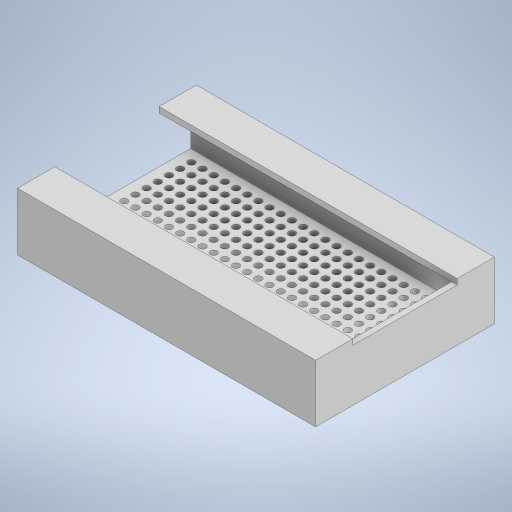
# Autodesk Inventor part: support batterie
Saved by Autodesk Inventor 2024 (Build 280153000, 153)
## iProperties
Created: 2024-02-10
Part Number: support batterie
Material: Generic
Document SubType Name: Modeling
Designer: Pooo
Density: 1 g/cm^3
Appearance: Default
Author: Pooo
Autodesk Inventor part; units mm, degrees
ref_plane "YZ Plane" through (0, 0, 0) normal (1, 0, 0) x (0, 1, 0)
ref_plane "XZ Plane" through (0, 0, 0) normal (0, 1, 0) x (-1, 0, 0)
ref_plane "XY Plane" through (0, 0, 0) normal (0, 0, 1) x (1, 0, 0)
sketch "Sketch1" plane through (0, 0, 0) normal (0, 1, 0) x (-1, 0, 0)
  point P0 (0, 0)
sketch "Sketch2" plane through (0, 0, 0) normal (0, 1, 0) x (-1, 0, 0)
  line L0 (43.1586, 43.7586) -> (-113.8414, 43.7586)
  line L1 (-113.8414, 43.7586) -> (-113.8414, -46.2414)
  line L2 (-113.8414, -46.2414) -> (43.1586, -46.2414)
  line L3 (43.1586, -46.2414) -> (43.1586, 43.7586)
  line L4 (43.1586, -46.2414) -> (-113.8414, -46.2414)
  line L5 (-113.8414, -46.2414) -> (-113.8414, -49.2414)
  line L6 (-113.8414, -49.2414) -> (43.1586, -49.2414)
  line L7 (43.1586, -49.2414) -> (43.1586, -46.2414)
  line L8 (43.1586, 43.7586) -> (-113.8414, 43.7586)
  line L9 (-113.8414, 43.7586) -> (-113.8414, 46.7586)
  line L10 (-113.8414, 46.7586) -> (43.1586, 46.7586)
  line L11 (43.1586, 46.7586) -> (43.1586, 43.7586)
  line L12 (-113.8414, 46.7586) -> (-116.8414, 46.7586)
  line L13 (-116.8414, 46.7586) -> (-116.8414, -49.2414)
  line L14 (-116.8414, -49.2414) -> (-113.8414, -49.2414)
  line L15 (-113.8414, -49.2414) -> (-113.8414, 46.7586)
  point P0 (0, 0)
  dimension "d0" = 90
  dimension "d1" = 157
  dimension "d2" = 3
  dimension "d3" = 3
  dimension "d4" = 3
  constraints: 32 end point, 8 parallel, 4 horizontal, 4 perpendicular
  measures "d0" distance of L2.end L0.start
  measures "d1" distance of L1.end L2.end
  measures "d2" distance of L4.end L5.end
  measures "d3" distance of L8.end L9.end
  measures "d4" distance of L14.end L13.end
extrude "Extrusion1" add sketch "Sketch2" along normal blind 3
sketch "Sketch3" plane through (0, 3, 0) normal (0, 1, 0) x (1, 0, 0)
  line L0 (-43.1586, -46.7586) -> (116.8414, -46.7586) projected
  line L1 (116.8414, -46.7586) -> (116.8414, 49.2414) projected
  line L2 (-43.1586, -46.7586) -> (116.8414, -46.7586)
  line L3 (116.8414, -46.7586) -> (116.8414, -43.7586)
  line L4 (116.8414, -43.7586) -> (-43.1586, -43.7586)
  line L5 (-43.1586, -43.7586) -> (-43.1586, -46.7586)
  line L6 (116.8414, 49.2414) -> (-43.1586, 49.2414) projected
  line L7 (-43.1586, 49.2414) -> (116.8414, 49.2414)
  line L8 (116.8414, 49.2414) -> (116.8414, 46.2414)
  line L9 (116.8414, 46.2414) -> (-43.1586, 46.2414)
  line L10 (-43.1586, 46.2414) -> (-43.1586, 49.2414)
  line L11 (116.8414, -43.7586) -> (113.8414, -43.7586)
  line L12 (113.8414, -43.7586) -> (113.8414, 46.2414)
  line L13 (113.8414, 46.2414) -> (116.8414, 46.2414)
  line L14 (116.8414, 46.2414) -> (116.8414, -43.7586)
  point P0 (0, 0)
  dimension "d7" = 3
  dimension "d8" = 3
  dimension "d9" = 3
  constraints: 24 end point, 6 parallel, 3 horizontal, 3 perpendicular, 3 point on line
  measures "d7" distance of L3.end L2.end
  measures "d8" distance of L7.end L8.end
  measures "d9" distance of L12.end L13.end
sketch "Sketch5" plane through (0, 3, 0) normal (0, 1, 0) x (1, 0, 0)
  circle A0 centre (-36.5125, -38.1) radius 1.85
  line L0 (-36.5125, -38.1) -> (-35.8777, -38.1)
  line L1 (-36.5125, -38.1) -> (-36.5125, -37.4601)
  circle A1 centre (-36.5125, -32.1) radius 1.85
  circle A2 centre (-36.5125, -26.1) radius 1.85
  circle A3 centre (-36.5125, -20.1) radius 1.85
  circle A4 centre (-36.5125, -14.1) radius 1.85
  circle A5 centre (-36.5125, -8.1) radius 1.85
  circle A6 centre (-36.5125, -2.1) radius 1.85
  circle A7 centre (-36.5125, 3.9) radius 1.85
  circle A8 centre (-36.5125, 9.9) radius 1.85
  circle A9 centre (-36.5125, 15.9) radius 1.85
  circle A10 centre (-36.5125, 21.9) radius 1.85
  circle A11 centre (-36.5125, 27.9) radius 1.85
  circle A12 centre (-36.5125, 33.9) radius 1.85
  circle A13 centre (-36.5125, 39.9) radius 1.85
  circle A14 centre (-30.5125, -38.1) radius 1.85
  circle A15 centre (-30.5125, -32.1) radius 1.85
  circle A16 centre (-30.5125, -26.1) radius 1.85
  circle A17 centre (-30.5125, -20.1) radius 1.85
  circle A18 centre (-30.5125, -14.1) radius 1.85
  circle A19 centre (-30.5125, -8.1) radius 1.85
  circle A20 centre (-30.5125, -2.1) radius 1.85
  circle A21 centre (-30.5125, 3.9) radius 1.85
  circle A22 centre (-30.5125, 9.9) radius 1.85
  circle A23 centre (-30.5125, 15.9) radius 1.85
  circle A24 centre (-30.5125, 21.9) radius 1.85
  circle A25 centre (-30.5125, 27.9) radius 1.85
  circle A26 centre (-30.5125, 33.9) radius 1.85
  circle A27 centre (-30.5125, 39.9) radius 1.85
  circle A28 centre (-24.5125, -38.1) radius 1.85
  circle A29 centre (-24.5125, -32.1) radius 1.85
  circle A30 centre (-24.5125, -26.1) radius 1.85
  circle A31 centre (-24.5125, -20.1) radius 1.85
  circle A32 centre (-24.5125, -14.1) radius 1.85
  circle A33 centre (-24.5125, -8.1) radius 1.85
  circle A34 centre (-24.5125, -2.1) radius 1.85
  circle A35 centre (-24.5125, 3.9) radius 1.85
  circle A36 centre (-24.5125, 9.9) radius 1.85
  circle A37 centre (-24.5125, 15.9) radius 1.85
  circle A38 centre (-24.5125, 21.9) radius 1.85
  circle A39 centre (-24.5125, 27.9) radius 1.85
  circle A40 centre (-24.5125, 33.9) radius 1.85
  circle A41 centre (-24.5125, 39.9) radius 1.85
  circle A42 centre (-18.5125, -38.1) radius 1.85
  circle A43 centre (-18.5125, -32.1) radius 1.85
  circle A44 centre (-18.5125, -26.1) radius 1.85
  circle A45 centre (-18.5125, -20.1) radius 1.85
  circle A46 centre (-18.5125, -14.1) radius 1.85
  circle A47 centre (-18.5125, -8.1) radius 1.85
  circle A48 centre (-18.5125, -2.1) radius 1.85
  circle A49 centre (-18.5125, 3.9) radius 1.85
  circle A50 centre (-18.5125, 9.9) radius 1.85
  circle A51 centre (-18.5125, 15.9) radius 1.85
  circle A52 centre (-18.5125, 21.9) radius 1.85
  circle A53 centre (-18.5125, 27.9) radius 1.85
  circle A54 centre (-18.5125, 33.9) radius 1.85
  circle A55 centre (-18.5125, 39.9) radius 1.85
  circle A56 centre (-12.5125, -38.1) radius 1.85
  circle A57 centre (-12.5125, -32.1) radius 1.85
  circle A58 centre (-12.5125, -26.1) radius 1.85
  circle A59 centre (-12.5125, -20.1) radius 1.85
  circle A60 centre (-12.5125, -14.1) radius 1.85
  circle A61 centre (-12.5125, -8.1) radius 1.85
  circle A62 centre (-12.5125, -2.1) radius 1.85
  circle A63 centre (-12.5125, 3.9) radius 1.85
  circle A64 centre (-12.5125, 9.9) radius 1.85
  circle A65 centre (-12.5125, 15.9) radius 1.85
  circle A66 centre (-12.5125, 21.9) radius 1.85
  circle A67 centre (-12.5125, 27.9) radius 1.85
  circle A68 centre (-12.5125, 33.9) radius 1.85
  circle A69 centre (-12.5125, 39.9) radius 1.85
  circle A70 centre (-6.5125, -38.1) radius 1.85
  circle A71 centre (-6.5125, -32.1) radius 1.85
  circle A72 centre (-6.5125, -26.1) radius 1.85
  circle A73 centre (-6.5125, -20.1) radius 1.85
  circle A74 centre (-6.5125, -14.1) radius 1.85
  circle A75 centre (-6.5125, -8.1) radius 1.85
  circle A76 centre (-6.5125, -2.1) radius 1.85
  circle A77 centre (-6.5125, 3.9) radius 1.85
  circle A78 centre (-6.5125, 9.9) radius 1.85
  circle A79 centre (-6.5125, 15.9) radius 1.85
  circle A80 centre (-6.5125, 21.9) radius 1.85
  circle A81 centre (-6.5125, 27.9) radius 1.85
  circle A82 centre (-6.5125, 33.9) radius 1.85
  circle A83 centre (-6.5125, 39.9) radius 1.85
  circle A84 centre (-0.5125, -38.1) radius 1.85
  circle A85 centre (-0.5125, -32.1) radius 1.85
  circle A86 centre (-0.5125, -26.1) radius 1.85
  circle A87 centre (-0.5125, -20.1) radius 1.85
  circle A88 centre (-0.5125, -14.1) radius 1.85
  circle A89 centre (-0.5125, -8.1) radius 1.85
  circle A90 centre (-0.5125, -2.1) radius 1.85
  circle A91 centre (-0.5125, 3.9) radius 1.85
  circle A92 centre (-0.5125, 9.9) radius 1.85
  circle A93 centre (-0.5125, 15.9) radius 1.85
  circle A94 centre (-0.5125, 21.9) radius 1.85
  circle A95 centre (-0.5125, 27.9) radius 1.85
  circle A96 centre (-0.5125, 33.9) radius 1.85
  circle A97 centre (-0.5125, 39.9) radius 1.85
  circle A98 centre (5.4875, -38.1) radius 1.85
  circle A99 centre (5.4875, -32.1) radius 1.85
  circle A100 centre (5.4875, -26.1) radius 1.85
  circle A101 centre (5.4875, -20.1) radius 1.85
  circle A102 centre (5.4875, -14.1) radius 1.85
  circle A103 centre (5.4875, -8.1) radius 1.85
  circle A104 centre (5.4875, -2.1) radius 1.85
  circle A105 centre (5.4875, 3.9) radius 1.85
  circle A106 centre (5.4875, 9.9) radius 1.85
  circle A107 centre (5.4875, 15.9) radius 1.85
  circle A108 centre (5.4875, 21.9) radius 1.85
  circle A109 centre (5.4875, 27.9) radius 1.85
  circle A110 centre (5.4875, 33.9) radius 1.85
  circle A111 centre (5.4875, 39.9) radius 1.85
  circle A112 centre (11.4875, -38.1) radius 1.85
  circle A113 centre (11.4875, -32.1) radius 1.85
  circle A114 centre (11.4875, -26.1) radius 1.85
  circle A115 centre (11.4875, -20.1) radius 1.85
  circle A116 centre (11.4875, -14.1) radius 1.85
  circle A117 centre (11.4875, -8.1) radius 1.85
  circle A118 centre (11.4875, -2.1) radius 1.85
  circle A119 centre (11.4875, 3.9) radius 1.85
  circle A120 centre (11.4875, 9.9) radius 1.85
  circle A121 centre (11.4875, 15.9) radius 1.85
  circle A122 centre (11.4875, 21.9) radius 1.85
  circle A123 centre (11.4875, 27.9) radius 1.85
  circle A124 centre (11.4875, 33.9) radius 1.85
  circle A125 centre (11.4875, 39.9) radius 1.85
  circle A126 centre (17.4875, -38.1) radius 1.85
  circle A127 centre (17.4875, -32.1) radius 1.85
  circle A128 centre (17.4875, -26.1) radius 1.85
  circle A129 centre (17.4875, -20.1) radius 1.85
  circle A130 centre (17.4875, -14.1) radius 1.85
  circle A131 centre (17.4875, -8.1) radius 1.85
  circle A132 centre (17.4875, -2.1) radius 1.85
  circle A133 centre (17.4875, 3.9) radius 1.85
  circle A134 centre (17.4875, 9.9) radius 1.85
  circle A135 centre (17.4875, 15.9) radius 1.85
  circle A136 centre (17.4875, 21.9) radius 1.85
  circle A137 centre (17.4875, 27.9) radius 1.85
  circle A138 centre (17.4875, 33.9) radius 1.85
  circle A139 centre (17.4875, 39.9) radius 1.85
  circle A140 centre (23.4875, -38.1) radius 1.85
  circle A141 centre (23.4875, -32.1) radius 1.85
  circle A142 centre (23.4875, -26.1) radius 1.85
  circle A143 centre (23.4875, -20.1) radius 1.85
  circle A144 centre (23.4875, -14.1) radius 1.85
  circle A145 centre (23.4875, -8.1) radius 1.85
  circle A146 centre (23.4875, -2.1) radius 1.85
  circle A147 centre (23.4875, 3.9) radius 1.85
  circle A148 centre (23.4875, 9.9) radius 1.85
  circle A149 centre (23.4875, 15.9) radius 1.85
  circle A150 centre (23.4875, 21.9) radius 1.85
  circle A151 centre (23.4875, 27.9) radius 1.85
  circle A152 centre (23.4875, 33.9) radius 1.85
  circle A153 centre (23.4875, 39.9) radius 1.85
  circle A154 centre (29.4875, -38.1) radius 1.85
  circle A155 centre (29.4875, -32.1) radius 1.85
  circle A156 centre (29.4875, -26.1) radius 1.85
  circle A157 centre (29.4875, -20.1) radius 1.85
  circle A158 centre (29.4875, -14.1) radius 1.85
  circle A159 centre (29.4875, -8.1) radius 1.85
  circle A160 centre (29.4875, -2.1) radius 1.85
  circle A161 centre (29.4875, 3.9) radius 1.85
  circle A162 centre (29.4875, 9.9) radius 1.85
  circle A163 centre (29.4875, 15.9) radius 1.85
  circle A164 centre (29.4875, 21.9) radius 1.85
  circle A165 centre (29.4875, 27.9) radius 1.85
  circle A166 centre (29.4875, 33.9) radius 1.85
  circle A167 centre (29.4875, 39.9) radius 1.85
  circle A168 centre (35.4875, -38.1) radius 1.85
  circle A169 centre (35.4875, -32.1) radius 1.85
  circle A170 centre (35.4875, -26.1) radius 1.85
  circle A171 centre (35.4875, -20.1) radius 1.85
  circle A172 centre (35.4875, -14.1) radius 1.85
  circle A173 centre (35.4875, -8.1) radius 1.85
  circle A174 centre (35.4875, -2.1) radius 1.85
  circle A175 centre (35.4875, 3.9) radius 1.85
  circle A176 centre (35.4875, 9.9) radius 1.85
  circle A177 centre (35.4875, 15.9) radius 1.85
  circle A178 centre (35.4875, 21.9) radius 1.85
  circle A179 centre (35.4875, 27.9) radius 1.85
  circle A180 centre (35.4875, 33.9) radius 1.85
  circle A181 centre (35.4875, 39.9) radius 1.85
  circle A182 centre (41.4875, -38.1) radius 1.85
  circle A183 centre (41.4875, -32.1) radius 1.85
  circle A184 centre (41.4875, -26.1) radius 1.85
  circle A185 centre (41.4875, -20.1) radius 1.85
  circle A186 centre (41.4875, -14.1) radius 1.85
  circle A187 centre (41.4875, -8.1) radius 1.85
  circle A188 centre (41.4875, -2.1) radius 1.85
  circle A189 centre (41.4875, 3.9) radius 1.85
  circle A190 centre (41.4875, 9.9) radius 1.85
  circle A191 centre (41.4875, 15.9) radius 1.85
  circle A192 centre (41.4875, 21.9) radius 1.85
  circle A193 centre (41.4875, 27.9) radius 1.85
  circle A194 centre (41.4875, 33.9) radius 1.85
  circle A195 centre (41.4875, 39.9) radius 1.85
  circle A196 centre (47.4875, -38.1) radius 1.85
  circle A197 centre (47.4875, -32.1) radius 1.85
  circle A198 centre (47.4875, -26.1) radius 1.85
  circle A199 centre (47.4875, -20.1) radius 1.85
  circle A200 centre (47.4875, -14.1) radius 1.85
  circle A201 centre (47.4875, -8.1) radius 1.85
  circle A202 centre (47.4875, -2.1) radius 1.85
  circle A203 centre (47.4875, 3.9) radius 1.85
  circle A204 centre (47.4875, 9.9) radius 1.85
  circle A205 centre (47.4875, 15.9) radius 1.85
  circle A206 centre (47.4875, 21.9) radius 1.85
  circle A207 centre (47.4875, 27.9) radius 1.85
  circle A208 centre (47.4875, 33.9) radius 1.85
  circle A209 centre (47.4875, 39.9) radius 1.85
  circle A210 centre (53.4875, -38.1) radius 1.85
  circle A211 centre (53.4875, -32.1) radius 1.85
  circle A212 centre (53.4875, -26.1) radius 1.85
  circle A213 centre (53.4875, -20.1) radius 1.85
  circle A214 centre (53.4875, -14.1) radius 1.85
  circle A215 centre (53.4875, -8.1) radius 1.85
  circle A216 centre (53.4875, -2.1) radius 1.85
  circle A217 centre (53.4875, 3.9) radius 1.85
  circle A218 centre (53.4875, 9.9) radius 1.85
  circle A219 centre (53.4875, 15.9) radius 1.85
  circle A220 centre (53.4875, 21.9) radius 1.85
  circle A221 centre (53.4875, 27.9) radius 1.85
  circle A222 centre (53.4875, 33.9) radius 1.85
  circle A223 centre (53.4875, 39.9) radius 1.85
  circle A224 centre (59.4875, -38.1) radius 1.85
  circle A225 centre (59.4875, -32.1) radius 1.85
  circle A226 centre (59.4875, -26.1) radius 1.85
  circle A227 centre (59.4875, -20.1) radius 1.85
  circle A228 centre (59.4875, -14.1) radius 1.85
  circle A229 centre (59.4875, -8.1) radius 1.85
  circle A230 centre (59.4875, -2.1) radius 1.85
  circle A231 centre (59.4875, 3.9) radius 1.85
  circle A232 centre (59.4875, 9.9) radius 1.85
  circle A233 centre (59.4875, 15.9) radius 1.85
  circle A234 centre (59.4875, 21.9) radius 1.85
  circle A235 centre (59.4875, 27.9) radius 1.85
  circle A236 centre (59.4875, 33.9) radius 1.85
  circle A237 centre (59.4875, 39.9) radius 1.85
  circle A238 centre (65.4875, -38.1) radius 1.85
  circle A239 centre (65.4875, -32.1) radius 1.85
  circle A240 centre (65.4875, -26.1) radius 1.85
  circle A241 centre (65.4875, -20.1) radius 1.85
  circle A242 centre (65.4875, -14.1) radius 1.85
  circle A243 centre (65.4875, -8.1) radius 1.85
  circle A244 centre (65.4875, -2.1) radius 1.85
  circle A245 centre (65.4875, 3.9) radius 1.85
  circle A246 centre (65.4875, 9.9) radius 1.85
  circle A247 centre (65.4875, 15.9) radius 1.85
  circle A248 centre (65.4875, 21.9) radius 1.85
  circle A249 centre (65.4875, 27.9) radius 1.85
  circle A250 centre (65.4875, 33.9) radius 1.85
  circle A251 centre (65.4875, 39.9) radius 1.85
  circle A252 centre (71.4875, -38.1) radius 1.85
  circle A253 centre (71.4875, -32.1) radius 1.85
  circle A254 centre (71.4875, -26.1) radius 1.85
  circle A255 centre (71.4875, -20.1) radius 1.85
  circle A256 centre (71.4875, -14.1) radius 1.85
  circle A257 centre (71.4875, -8.1) radius 1.85
  circle A258 centre (71.4875, -2.1) radius 1.85
  circle A259 centre (71.4875, 3.9) radius 1.85
  circle A260 centre (71.4875, 9.9) radius 1.85
  circle A261 centre (71.4875, 15.9) radius 1.85
  circle A262 centre (71.4875, 21.9) radius 1.85
  circle A263 centre (71.4875, 27.9) radius 1.85
  circle A264 centre (71.4875, 33.9) radius 1.85
  circle A265 centre (71.4875, 39.9) radius 1.85
  circle A266 centre (77.4875, -38.1) radius 1.85
  circle A267 centre (77.4875, -32.1) radius 1.85
  circle A268 centre (77.4875, -26.1) radius 1.85
  circle A269 centre (77.4875, -20.1) radius 1.85
  circle A270 centre (77.4875, -14.1) radius 1.85
  circle A271 centre (77.4875, -8.1) radius 1.85
  circle A272 centre (77.4875, -2.1) radius 1.85
  circle A273 centre (77.4875, 3.9) radius 1.85
  circle A274 centre (77.4875, 9.9) radius 1.85
  circle A275 centre (77.4875, 15.9) radius 1.85
  circle A276 centre (77.4875, 21.9) radius 1.85
  circle A277 centre (77.4875, 27.9) radius 1.85
  circle A278 centre (77.4875, 33.9) radius 1.85
  circle A279 centre (77.4875, 39.9) radius 1.85
  circle A280 centre (83.4875, -38.1) radius 1.85
  circle A281 centre (83.4875, -32.1) radius 1.85
  circle A282 centre (83.4875, -26.1) radius 1.85
  circle A283 centre (83.4875, -20.1) radius 1.85
  circle A284 centre (83.4875, -14.1) radius 1.85
  circle A285 centre (83.4875, -8.1) radius 1.85
  circle A286 centre (83.4875, -2.1) radius 1.85
  circle A287 centre (83.4875, 3.9) radius 1.85
  circle A288 centre (83.4875, 9.9) radius 1.85
  circle A289 centre (83.4875, 15.9) radius 1.85
  circle A290 centre (83.4875, 21.9) radius 1.85
  circle A291 centre (83.4875, 27.9) radius 1.85
  circle A292 centre (83.4875, 33.9) radius 1.85
  circle A293 centre (83.4875, 39.9) radius 1.85
  circle A294 centre (89.4875, -38.1) radius 1.85
  circle A295 centre (89.4875, -32.1) radius 1.85
  circle A296 centre (89.4875, -26.1) radius 1.85
  circle A297 centre (89.4875, -20.1) radius 1.85
  circle A298 centre (89.4875, -14.1) radius 1.85
  circle A299 centre (89.4875, -8.1) radius 1.85
  circle A300 centre (89.4875, -2.1) radius 1.85
  circle A301 centre (89.4875, 3.9) radius 1.85
  circle A302 centre (89.4875, 9.9) radius 1.85
  circle A303 centre (89.4875, 15.9) radius 1.85
  circle A304 centre (89.4875, 21.9) radius 1.85
  circle A305 centre (89.4875, 27.9) radius 1.85
  circle A306 centre (89.4875, 33.9) radius 1.85
  circle A307 centre (89.4875, 39.9) radius 1.85
  circle A308 centre (95.4875, -38.1) radius 1.85
  circle A309 centre (95.4875, -32.1) radius 1.85
  circle A310 centre (95.4875, -26.1) radius 1.85
  circle A311 centre (95.4875, -20.1) radius 1.85
  circle A312 centre (95.4875, -14.1) radius 1.85
  circle A313 centre (95.4875, -8.1) radius 1.85
  circle A314 centre (95.4875, -2.1) radius 1.85
  circle A315 centre (95.4875, 3.9) radius 1.85
  circle A316 centre (95.4875, 9.9) radius 1.85
  circle A317 centre (95.4875, 15.9) radius 1.85
  circle A318 centre (95.4875, 21.9) radius 1.85
  circle A319 centre (95.4875, 27.9) radius 1.85
  circle A320 centre (95.4875, 33.9) radius 1.85
  circle A321 centre (95.4875, 39.9) radius 1.85
  circle A322 centre (101.4875, -38.1) radius 1.85
  circle A323 centre (101.4875, -32.1) radius 1.85
  circle A324 centre (101.4875, -26.1) radius 1.85
  circle A325 centre (101.4875, -20.1) radius 1.85
  circle A326 centre (101.4875, -14.1) radius 1.85
  circle A327 centre (101.4875, -8.1) radius 1.85
  circle A328 centre (101.4875, -2.1) radius 1.85
  circle A329 centre (101.4875, 3.9) radius 1.85
  circle A330 centre (101.4875, 9.9) radius 1.85
  circle A331 centre (101.4875, 15.9) radius 1.85
  circle A332 centre (101.4875, 21.9) radius 1.85
  circle A333 centre (101.4875, 27.9) radius 1.85
  circle A334 centre (101.4875, 33.9) radius 1.85
  circle A335 centre (101.4875, 39.9) radius 1.85
  circle A336 centre (107.4875, -38.1) radius 1.85
  circle A337 centre (107.4875, -32.1) radius 1.85
  circle A338 centre (107.4875, -26.1) radius 1.85
  circle A339 centre (107.4875, -20.1) radius 1.85
  circle A340 centre (107.4875, -14.1) radius 1.85
  circle A341 centre (107.4875, -8.1) radius 1.85
  circle A342 centre (107.4875, -2.1) radius 1.85
  circle A343 centre (107.4875, 3.9) radius 1.85
  circle A344 centre (107.4875, 9.9) radius 1.85
  circle A345 centre (107.4875, 15.9) radius 1.85
  circle A346 centre (107.4875, 21.9) radius 1.85
  circle A347 centre (107.4875, 27.9) radius 1.85
  circle A348 centre (107.4875, 33.9) radius 1.85
  circle A349 centre (107.4875, 39.9) radius 1.85
  point P0 (0, 0)
  dimension "d10" = 3.7
  dimension "d13" = 6
  dimension "d16" = 6
  constraints: 350 centre point, 4 end point, 2 horizontal, 2 vertical, 698 other
  measures "d10" diameter of A0
  measures "d13" distance of L0.start A1.centre
  measures "d16" distance of L0.start A14.centre
extrude "Extrusion2" cut sketch "Sketch5" against normal blind 4
extrude "Extrusion3" add sketch "Sketch3" along normal blind 25
sketch "Sketch8" plane through (0, 28, 0) normal (0, 1, 0) x (1, 0, 0)
  line L0 (116.8414, -46.7586) -> (116.8414, 49.2414) projected
  line L1 (-43.1586, 49.2414) -> (116.8414, 49.2414)
  line L2 (116.8414, 49.2414) -> (116.8414, 29.2414)
  line L3 (116.8414, 29.2414) -> (-43.1586, 29.2414)
  line L4 (-43.1586, 29.2414) -> (-43.1586, 49.2414)
  line L5 (116.8414, -46.7586) -> (-43.1586, -46.7586)
  line L6 (-43.1586, -46.7586) -> (-43.1586, -26.7586)
  line L7 (-43.1586, -26.7586) -> (116.8414, -26.7586)
  line L8 (116.8414, -26.7586) -> (116.8414, -46.7586)
  point P0 (0, 0)
  dimension "d23" = 20
  dimension "d24" = 20
  constraints: 16 end point, 4 parallel, 2 horizontal, 2 perpendicular, 2 point on line
  measures "d23" distance of L1.end L2.end
  measures "d24" distance of L5.end L6.end
extrude "Extrusion4" add sketch "Sketch8" along normal blind 3
body "Solid1"
